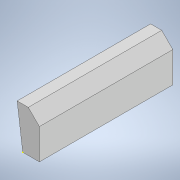
# Autodesk Inventor part: outside-join-half
Saved by Autodesk Inventor 2021 (Build 250183000, 183)
## iProperties
Created: 2020-12-10
Part Number: outside-join-half
Material: Generic
Document SubType Name: Modeling
Designer: Luke Kamols
Density: 1 g/cm^3
Appearance: Default
Author: Luke Kamols
Autodesk Inventor part; units mm, degrees
ref_plane "YZ Plane" through (0, 0, 0) normal (1, 0, 0) x (0, 1, 0)
ref_plane "XZ Plane" through (0, 0, 0) normal (0, 1, 0) x (-1, 0, 0)
ref_plane "XY Plane" through (0, 0, 0) normal (0, 0, 1) x (1, 0, 0)
sketch "Sketch1" plane through (0, 0, 0) normal (0, 0, 1) x (1, 0, 0)
  line L0 (0, 0) -> (6, 0)
  line L1 (6, 0) -> (6, 11)
  line L2 (0, 15) -> (2, 15)
  line L3 (2, 15) -> (6, 11)
  line L4 (0, 15) -> (-2, 15)
  line L5 (-2, 15) -> (0, 0)
  dimension "d0" = 6
  dimension "d1" = 11
  dimension "d2" = 15
  dimension "d4" = 2
  dimension "d5" = 2
  constraints: 12 end point, 3 horizontal, 1 perpendicular
  measures "d0" distance of L0.start L0.end
  measures "d1" distance of L0.end L1.end
  measures "d2" distance of L0.start L2.start
  measures "d4" distance of L2.start L2.end
  measures "d5" distance of L2.start L4.end
extrude "Extrusion1" add sketch "Sketch1" along normal blind 10.4
sketch "Sketch2" plane through (0, 0, 10.4) normal (0, 0, 1) x (1, 0, 0)
  line L0 (6, 0) -> (6, 11) projected
  line L1 (6, 0) -> (6, 11)
  line L2 (6, 11) -> (2, 15) projected
  line L3 (6, 11) -> (2, 15)
  line L4 (-2, 15) -> (0, 0) projected
  line L5 (2, 15) -> (-2, 15)
  line L6 (0, 0) -> (6, 0) projected
  line L7 (6, 0) -> (3, 0)
  line L8 (0, 11) -> (3, 0)
  line L9 (-3, 0) -> (0, 11)
  line L10 (-6, 11) -> (-2, 15)
  line L11 (-5, 0) -> (-6, 4)
  line L12 (-3, 0) -> (-5, 0)
  line L13 (-6, 4) -> (-6, 11)
  line L14 (-6, 11) -> (-5.6, 11)
  line L15 (-5.6, 11) -> (-5.6, 11.4)
  line L16 (-5.6, 11) -> (-5.6, 4)
  line L17 (-5, 0) -> (-4.6, 0)
  line L18 (-4.6, 0) -> (-5.6, 4)
  line L19 (-3, 0) -> (-3.4, 0)
  line L20 (0, 11) -> (0, 11.4)
  line L21 (0, 11.4) -> (-3.4, 0)
  line L22 (3, 0) -> (3.4, 0)
  line L23 (3.4, 0) -> (0, 11.4)
  point P0 (-0.9851, 7.3881)
  dimension "d9" = 3
  dimension "d45" = 0.4
  dimension "d46" = 0.4
  dimension "d47" = 0.4
  dimension "d48" = 0.4
  constraints: 40 end point, 4 point on line, 3 horizontal, 3 vertical, 2 collinear, 1 midpoint, 1 perpendicular
  measures "d9" distance of L4.end L9.start
  measures "d45" distance of L10.start L14.end
  measures "d46" distance of L11.start L17.end
  measures "d47" distance of L9.start L19.end
  measures "d48" distance of L7.end L22.end
extrude "Extrusion2" add sketch "Sketch2" along normal blind 27.2 contours L6 L23 L21 L4 L5 L2 L0 | L4 L21 L12 L18 L16 L15 L10
sketch "Sketch3" plane through (0, 0, 37.6) normal (0, 0, 1) x (1, 0, 0)
  line L0 (-2, 15) -> (0, 0) projected
  line L1 (2, 15) -> (-2, 15) projected
  line L2 (6, 11) -> (2, 15) projected
  line L3 (6, 0) -> (6, 11) projected
  line L4 (0, 0) -> (6, 0) projected
extrude "Extrusion3" add sketch "Sketch3" along normal blind 10.4
sketch "Sketch6" plane through (6, 0, 0) normal (1, 0, 0) x (0, 0, -1)
  line L0 (0, 15) -> (0, 0) projected
  line L1 (0, 0) -> (-10.4, 0) projected
  line L2 (0, 0) -> (-10.4, 0)
  line L3 (-10.4, 15) -> (-10.4, 7.878) projected
  line L4 (0, 15) -> (-10.4, 15) projected
  line L5 (-10.4, 7.878) -> (-10.4, 0) projected
  line L6 (-10.4, 0) -> (-10.4, 0)
  line L7 (-10.4, 0) -> (-10.4, 15)
  line L8 (-10.4, 15) -> (-8.4, 15)
  line L9 (-8.4, 15) -> (-10.4, 0)
  point P0 (-10.4, 7.3881)
  dimension "d19" = 15
  dimension "d38" = 15
  dimension "d39" = 2
  constraints: 10 end point, 1 collinear, 1 perpendicular, 1 point on line
  measures "d19" distance of L1.end L3.start
  measures "d38" distance of L6.end L7.end
  measures "d39" distance of L7.end L8.end
extrude "Extrusion4" cut sketch "Sketch6" against normal blind 33.8125 contours L9 L5 L3 L4
sketch "Sketch7" plane through (0, 0, 10.4) normal (0, 0, -1) x (-1, 0, 0)
  line L0 (3.4, 0) -> (0, 11.4) projected
  line L1 (4.6, 0) -> (3.4, 0) projected
  line L2 (5.6, 4) -> (4.6, 0) projected
  line L3 (5.6, 11.4) -> (5.6, 4) projected
  line L4 (2, 15) -> (5.6, 11.4) projected
  line L5 (-2, 15) -> (2, 15) projected
  line L6 (-6, 11) -> (-2, 15) projected
  line L7 (-6, 0) -> (-6, 11) projected
  line L8 (-3.4, 0) -> (-6, 0) projected
  line L9 (-3.4, 0) -> (0, 11.4) projected
extrude "Extrusion5" add sketch "Sketch7" along normal up to surface surface through (6, 15, 8.4) normal (0, -0.1321637, -0.9912279)
sketch "Sketch8" plane through (0, 0, 37.6) normal (0, 0, -1) x (-1, 0, 0)
  line L0 (0, 0) -> (-3.4, 0) projected
  line L1 (1.0504, 7.878) -> (0, 0) projected
  line L2 (0, 11.4) -> (-3.4, 0) projected
  line L3 (1.0504, 7.878) -> (0, 11.4) projected
extrude "Extrusion6" cut sketch "Sketch8" along normal blind 30 and the other way blind 2
sketch "Sketch10" plane through (6, 0, 0) normal (1, 0, 0) x (0, 0, -1)
  line L0 (0, 11) -> (-48, 11) projected
  line L1 (-48, 0) -> (-48, 11) projected
  line L2 (0, 0) -> (-48, 0) projected
  line L3 (0, 0) -> (0, 11) projected
  line L4 (-48, 0) -> (-37.6, 0)
  line L5 (-39.6, 0) -> (-7.6, 0) projected
  line L6 (-8.4, 15) -> (-37.6, 15) projected
  line L7 (-37.6, 0) -> (-37.6, 15)
  line L8 (-37.6, 15) -> (-39.6, 15)
  line L9 (-37.6, 15) -> (-48, 15) projected
  line L10 (-37.6, 4) -> (-37.6, 0) projected
  line L11 (-39.6, 15) -> (-37.6, 0)
  point P0 (-10.4, 15)
  point P1 (-10.4, 15)
  dimension "d49" = 2
  constraints: 8 end point, 2 point on line, 1 perpendicular
  measures "d49" distance of L6.end L8.end
extrude "Extrusion7" cut sketch "Sketch10" against normal blind 17.625 contours L7 L11 L0 | L0 L11 L8 L7
sketch "Sketch12" plane through (0, 0, 37.6) normal (0, 0, 1) x (1, 0, 0)
  line L0 (-2, 15) -> (-5.6, 11.4) projected
  line L1 (-4.6, 0) -> (-3.4, 0) projected
  line L2 (-5.6, 11.4) -> (-5.6, 4) projected
  line L3 (-5.6, 4) -> (-4.6, 0) projected
  line L4 (-3.4, 0) -> (0, 11.4) projected
  line L5 (3.4, 0) -> (0, 11.4) projected
  line L6 (3.4, 0) -> (6, 0) projected
  line L7 (6, 11) -> (6, 0) projected
  line L8 (2, 15) -> (6, 11) projected
  line L9 (-2, 15) -> (2, 15) projected
  point P0 (0, 0)
extrude "Extrusion8" add sketch "Sketch12" along normal up to surface surface through (6, 0, 37.6) normal (0, -0.1321637, 0.9912279)
sketch "Sketch14" plane through (0, 0, 48) normal (0, 0, 1) x (1, 0, 0)
  point P0 (0, 0)
body "Solid1"
